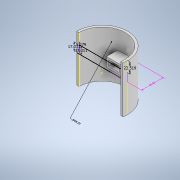
# Autodesk Inventor part: airframe
Saved by Autodesk Inventor 2022 (Build 260153000, 153)
## iProperties
Created: 2021-07-29
Part Number: airframe
Material: Generic
Document SubType Name: Modeling
Designer: WASHINGTON
Density: 1 g/cm^3
Appearance: Default
Author: WASHINGTON
Autodesk Inventor part; units mm, degrees
ref_plane "YZ Plane" through (0, 0, 0) normal (1, 0, 0) x (0, 1, 0)
ref_plane "XZ Plane" through (0, 0, 0) normal (0, 1, 0) x (-1, 0, 0)
ref_plane "XY Plane" through (0, 0, 0) normal (0, 0, 1) x (1, 0, 0)
sketch "Sketch1" plane through (0, 0, 0) normal (0, 1, 0) x (-1, 0, 0)
  arc A0 (-48.5586, 8.5622) -> (49.3077, 0) centre (0, 0) ccw construction
  line L0 (-25, -42.5) -> (25, -42.5) construction
  line L1 (25, -42.5) -> (25, 42.5) construction
  line L2 (25, 42.5) -> (-25, 42.5) construction
  line L3 (-25, -42.5) -> (25, 42.5) construction
  line L4 (25, -42.5) -> (-25, 42.5) construction
  arc A1 (-48.5586, 8.5622) -> (49.3077, 0) centre (0, 0) ccw
  arc A2 (-53.4827, 9.4304) -> (54.3077, 0) centre (0, 0) ccw
  line L5 (-48.5586, 8.5622) -> (-53.4827, 9.4304)
  line L6 (54.3077, 0) -> (49.3077, 0)
  dimension "d0" = 85
  dimension "d1" = 50
  dimension "d2" = 5
  dimension "d4" = 54.3077
  dimension "d5" = 59.535
  dimension "d6" = 170
  dimension "d7" = 42.5
  dimension "d8" = 0
  constraints: 14 end point, 6 point on circle, 3 centre point, 2 coincident, 2 horizontal, 2 midpoint, 1 concentric, 1 parallel, 1 perpendicular
  measures "d0" distance of L0.end L1.end
  measures "d1" distance of L0.start L0.end
  measures "d2" radial gap between concentric circles of A0 A2
  measures "d4" radius of A2
  measures "d5" angle of L6 L4
  measures "d6" angle of L6 L5
  measures "d7" distance between parallel lines of L6 L0
  measures "d8" distance from line of point (0, 0) L5
extrude "Extrusion1" add sketch "Sketch1" along normal mid plane 100
sketch "Sketch2" plane through (0, 0, 0) normal (1, 0, 0) x (0, 1, 0)
  point P0 (0, 0)
sketch "Sketch3" plane through (0, 0, 0) normal (0, 0, 1) x (1, 0, 0)
  line L0 (11.5, -6) -> (-11.5, -6)
  line L1 (-11.5, -6) -> (-11.5, 6)
  line L2 (-11.5, 6) -> (11.5, 6)
  line L3 (11.5, 6) -> (11.5, -6)
  line L4 (11.5, -6) -> (-11.5, 6) construction
  line L5 (-11.5, -6) -> (11.5, 6) construction
  line L6 (15.5, 10) -> (-15.5, 10)
  line L7 (-15.5, 10) -> (-15.5, -10)
  line L8 (-15.5, -10) -> (15.5, -10)
  line L9 (15.5, -10) -> (15.5, 10)
  point P0 (0, 0)
  dimension "d11" = 23
  dimension "d12" = 12
  dimension "d13" = 4
  constraints: 20 end point, 4 parallel, 2 midpoint, 2 perpendicular, 1 horizontal, 3 other
  measures "d11" distance of L1.end L2.end
  measures "d12" distance of L0.start L2.end
  measures "d13" distance between parallel lines of L2 L6
extrude "Extrusion2" add sketch "Sketch3" against normal up to next
sketch "Sketch4" plane through (0, 0, 0) normal (0, 0, 1) x (1, 0, 0)
  line L0 (15.5, 10) -> (-15.5, 10) projected
  line L1 (-15.5, -10) -> (15.5, -10)
  line L2 (15.5, -10) -> (15.5, 10)
  line L3 (15.5, 10) -> (-15.5, 10)
  line L4 (-15.5, 10) -> (-15.5, -10)
  line L5 (-15.5, -10) -> (15.5, 10) construction
  line L6 (15.5, -10) -> (-15.5, 10) construction
  point P0 (0, 0)
  point P1 (-15.5, 10)
  constraints: 12 end point, 2 midpoint, 2 parallel, 1 horizontal, 1 perpendicular
extrude "Extrusion3" cut sketch "Sketch4" against normal blind 25
sketch "Sketch5" plane through (0, 0, 0) normal (0, 1, 0) x (-1, 0, 0)
  point P0 (0, 0)
sketch "Sketch6" plane through (0, 0, 0) normal (0, 0, 1) x (1, 0, 0)
  line L0 (-49.3077, -50) -> (-49.3077, 50) projected
  line L1 (-49.3077, 32.7599) -> (-49.3077, 10.4691)
  line L2 (53.4827, -50) -> (53.4827, 50) projected
  line L3 (53.4827, 10.4691) -> (-53.8854, 10.4691)
  line L4 (-49.3077, 27.4805) -> (53.4827, 27.4805)
  line L5 (53.4827, 27.4805) -> (53.4827, 10.4691)
  line L6 (-49.3077, 10.4691) -> (-49.3077, 27.4805)
  line L7 (48.7697, 10.4691) -> (48.5586, 27.4805)
  line L8 (48.5586, -50) -> (48.5586, 50) projected
  point P0 (0, 0)
  dimension "d24" = 17.0114
  dimension "d25" = 22.5195
  dimension "d26" = 5.2794
  dimension "d27" = 17.0114
  constraints: 12 end point, 6 point on line, 1 horizontal, 1 parallel
  measures "d24" distance between parallel lines of L4 L3
  measures "d25" distance from line of L2.end L4
  measures "d26" distance from line of L1.start L4
  measures "d27" distance from line of L1.end L4
body "Solid1"
